Autodesk Inventor part; units mm, degrees
(part 10 of 11)
sketch "22" plane through (0, 0, 0) normal (0, 0, 1) x (1, 0, 0)
  line L0 (33.782, 19.812) -> (33.782, 30.7159)
  arc A0 (-2.032, 21.8669) -> (-2.032, 19.0271) centre (-2.032, 20.447) ccw
  arc A1 (-2.032, 19.0271) -> (-2.032, 21.8669) centre (-2.032, 20.447) ccw
  arc A2 (16.383, 40.2819) -> (16.383, 37.4421) centre (16.383, 38.862) ccw
  arc A3 (16.383, 37.4421) -> (16.383, 40.2819) centre (16.383, 38.862) ccw
  arc A4 (0.508, 19.8438) -> (0.508, 19.7803) centre (0.508, 19.812) ccw
  arc A5 (3.048, 19.7803) -> (3.048, 19.8438) centre (3.048, 19.812) ccw
  line L1 (0.508, 19.812) -> (3.048, 19.812)
  arc A6 (-0.7395, 21.1045) -> (-0.7845, 21.0595) centre (-0.762, 21.082) ccw
  arc A7 (0.4855, 19.7895) -> (0.5305, 19.8345) centre (0.508, 19.812) ccw
  line L2 (-0.762, 21.082) -> (0.508, 19.812)
  arc A8 (-2.0545, 19.8345) -> (-2.0095, 19.7895) centre (-2.032, 19.812) ccw
  arc A9 (-0.7395, 21.0595) -> (-0.7845, 21.1045) centre (-0.762, 21.082) ccw
  line L3 (-2.032, 19.812) -> (-0.762, 21.082)
  arc A10 (-0.7845, 18.5195) -> (-0.7395, 18.5645) centre (-0.762, 18.542) ccw
  arc A11 (-2.0095, 19.8345) -> (-2.0545, 19.7895) centre (-2.032, 19.812) ccw
  line L4 (-0.762, 18.542) -> (-2.032, 19.812)
  arc A12 (3.048, 18.5103) -> (3.048, 18.5738) centre (3.048, 18.542) ccw
  arc A13 (-0.762, 18.5738) -> (-0.762, 18.5102) centre (-0.762, 18.542) ccw
  line L5 (3.048, 18.542) -> (-0.762, 18.542)
  arc A14 (17.0498, 36.322) -> (16.9862, 36.322) centre (17.018, 36.322) ccw
  arc A15 (16.9862, 33.782) -> (17.0497, 33.782) centre (17.018, 33.782) ccw
  line L6 (17.018, 36.322) -> (17.018, 33.782)
  arc A16 (15.7705, 37.6145) -> (15.7255, 37.5695) centre (15.748, 37.592) ccw
  arc A17 (16.9955, 36.2995) -> (17.0405, 36.3445) centre (17.018, 36.322) ccw
  line L7 (15.748, 37.592) -> (17.018, 36.322)
  arc A18 (17.0405, 38.8395) -> (16.9955, 38.8845) centre (17.018, 38.862) ccw
  arc A19 (15.7255, 37.6145) -> (15.7705, 37.5695) centre (15.748, 37.592) ccw
  line L8 (17.018, 38.862) -> (15.748, 37.592)
  arc A20 (18.2655, 37.5695) -> (18.3105, 37.6145) centre (18.288, 37.592) ccw
  arc A21 (17.0405, 38.8845) -> (16.9955, 38.8395) centre (17.018, 38.862) ccw
  line L9 (18.288, 37.592) -> (17.018, 38.862)
  arc A22 (18.2563, 33.782) -> (18.3197, 33.782) centre (18.288, 33.782) ccw
  arc A23 (18.3198, 37.592) -> (18.2562, 37.592) centre (18.288, 37.592) ccw
  line L10 (18.288, 33.782) -> (18.288, 37.592)
  arc A24 (18.2563, 18.542) -> (18.3197, 18.542) centre (18.288, 18.542) ccw
  arc A25 (18.3197, 33.782) -> (18.2563, 33.782) centre (18.288, 33.782) ccw
  line L11 (18.288, 18.542) -> (18.288, 33.782)
  arc A26 (3.048, 18.5738) -> (3.048, 18.5103) centre (3.048, 18.542) ccw
  arc A27 (18.288, 18.5103) -> (18.288, 18.5738) centre (18.288, 18.542) ccw
  line L12 (3.048, 18.542) -> (18.288, 18.542)
  arc A28 (3.0162, 18.542) -> (3.0797, 18.542) centre (3.048, 18.542) ccw
  line L13 (3.048, 19.812) -> (3.048, 18.542)
  arc A29 (3.0797, 30.7159) -> (3.0162, 30.7159) centre (3.048, 30.7159) ccw
  arc A30 (3.0162, 19.812) -> (3.0797, 19.812) centre (3.048, 19.812) ccw
  line L14 (3.048, 30.7159) -> (3.048, 19.812)
  arc A31 (3.0162, 30.7159) -> (3.0797, 30.7159) centre (3.048, 30.7159) ccw
  line L15 (18.542, 3.048) -> (19.812, 3.048)
  arc A32 (19.812, 3.0162) -> (19.812, 3.0797) centre (19.812, 3.048) ccw
  arc A33 (18.542, 3.0797) -> (18.542, 3.0162) centre (18.542, 3.048) ccw
  line L16 (19.812, 3.048) -> (30.7159, 3.048)
  arc A34 (30.7159, 3.0162) -> (30.7159, 3.0797) centre (30.7159, 3.048) ccw
  arc A35 (19.812, 3.0797) -> (19.812, 3.0162) centre (19.812, 3.048) ccw
  arc A36 (6.1141, 33.7503) -> (6.1141, 33.8137) centre (6.1141, 33.782) ccw
  arc A37 (6.1141, 33.782) -> (3.048, 30.7159) centre (6.1141, 30.7159) ccw
  arc A38 (17.018, 33.7503) -> (17.018, 33.8137) centre (17.018, 33.782) ccw
  arc A39 (6.1141, 33.8137) -> (6.1141, 33.7503) centre (6.1141, 33.782) ccw
  line L17 (17.018, 33.782) -> (6.1141, 33.782)
  arc A40 (18.288, 33.7503) -> (18.288, 33.8137) centre (18.288, 33.782) ccw
  arc A41 (17.018, 33.8137) -> (17.018, 33.7503) centre (17.018, 33.782) ccw
  line L18 (18.288, 33.782) -> (17.018, 33.782)
  arc A42 (33.8137, 30.7159) -> (33.7503, 30.7159) centre (33.782, 30.7159) ccw
  arc A43 (20.447, 40.2819) -> (20.447, 37.4421) centre (20.447, 38.862) ccw
  arc A44 (20.447, 37.4421) -> (20.447, 40.2819) centre (20.447, 38.862) ccw
  arc A45 (38.862, 21.8669) -> (38.862, 19.0271) centre (38.862, 20.447) ccw
  arc A46 (38.862, 19.0271) -> (38.862, 21.8669) centre (38.862, 20.447) ccw
  arc A47 (19.8438, 36.322) -> (19.7803, 36.322) centre (19.812, 36.322) ccw
  arc A48 (19.7803, 33.782) -> (19.8438, 33.782) centre (19.812, 33.782) ccw
  line L19 (19.812, 36.322) -> (19.812, 33.782)
  arc A49 (21.1045, 37.5695) -> (21.0595, 37.6145) centre (21.082, 37.592) ccw
  arc A50 (19.7895, 36.3445) -> (19.8345, 36.2995) centre (19.812, 36.322) ccw
  line L20 (21.082, 37.592) -> (19.812, 36.322)
  arc A51 (19.8345, 38.8845) -> (19.7895, 38.8395) centre (19.812, 38.862) ccw
  arc A52 (21.0595, 37.5695) -> (21.1045, 37.6145) centre (21.082, 37.592) ccw
  line L21 (19.812, 38.862) -> (21.082, 37.592)
  arc A53 (18.5195, 37.6145) -> (18.5645, 37.5695) centre (18.542, 37.592) ccw
  arc A54 (19.8345, 38.8395) -> (19.7895, 38.8845) centre (19.812, 38.862) ccw
  line L22 (18.542, 37.592) -> (19.812, 38.862)
  arc A55 (18.5103, 33.782) -> (18.5738, 33.782) centre (18.542, 33.782) ccw
  arc A56 (18.5738, 37.592) -> (18.5102, 37.592) centre (18.542, 37.592) ccw
  line L23 (18.542, 33.782) -> (18.542, 37.592)
  arc A57 (36.322, 19.7803) -> (36.322, 19.8438) centre (36.322, 19.812) ccw
  arc A58 (33.782, 19.8438) -> (33.782, 19.7803) centre (33.782, 19.812) ccw
  line L24 (36.322, 19.812) -> (33.782, 19.812)
  arc A59 (37.6145, 21.0595) -> (37.5695, 21.1045) centre (37.592, 21.082) ccw
  arc A60 (36.2995, 19.8345) -> (36.3445, 19.7895) centre (36.322, 19.812) ccw
  line L25 (37.592, 21.082) -> (36.322, 19.812)
  arc A61 (38.8395, 19.7895) -> (38.8845, 19.8345) centre (38.862, 19.812) ccw
  arc A62 (37.6145, 21.1045) -> (37.5695, 21.0595) centre (37.592, 21.082) ccw
  line L26 (38.862, 19.812) -> (37.592, 21.082)
  arc A63 (37.5695, 18.5645) -> (37.6145, 18.5195) centre (37.592, 18.542) ccw
  arc A64 (33.7503, 19.812) -> (33.8137, 19.812) centre (33.782, 19.812) ccw
  arc A65 (38.8845, 19.7895) -> (38.8395, 19.8345) centre (38.862, 19.812) ccw
  line L27 (37.592, 18.542) -> (38.862, 19.812)
  arc A66 (33.782, 18.5738) -> (33.782, 18.5103) centre (33.782, 18.542) ccw
  arc A67 (37.592, 18.5102) -> (37.592, 18.5738) centre (37.592, 18.542) ccw
  line L28 (33.782, 18.542) -> (37.592, 18.542)
  arc A68 (18.542, 18.5738) -> (18.542, 18.5103) centre (18.542, 18.542) ccw
  arc A69 (33.782, 18.5103) -> (33.782, 18.5738) centre (33.782, 18.542) ccw
  line L29 (18.542, 18.542) -> (33.782, 18.542)
  arc A70 (18.5738, 33.782) -> (18.5103, 33.782) centre (18.542, 33.782) ccw
  arc A71 (18.5103, 18.542) -> (18.5738, 18.542) centre (18.542, 18.542) ccw
  line L30 (18.542, 33.782) -> (18.542, 18.542)
  arc A72 (19.812, 33.7503) -> (19.812, 33.8137) centre (19.812, 33.782) ccw
  arc A73 (18.542, 33.8137) -> (18.542, 33.7503) centre (18.542, 33.782) ccw
  line L31 (19.812, 33.782) -> (18.542, 33.782)
  arc A74 (30.7159, 33.7503) -> (30.7159, 33.8137) centre (30.7159, 33.782) ccw
  arc A75 (19.812, 33.8137) -> (19.812, 33.7503) centre (19.812, 33.782) ccw
  line L32 (30.7159, 33.782) -> (19.812, 33.782)
  arc A76 (30.7159, 33.8137) -> (30.7159, 33.7503) centre (30.7159, 33.782) ccw
  arc A77 (33.7503, 30.7159) -> (33.8137, 30.7159) centre (33.782, 30.7159) ccw
  arc A78 (33.782, 30.7159) -> (30.7159, 33.782) centre (30.7159, 30.7159) ccw
  arc A79 (3.0797, 19.812) -> (3.0162, 19.812) centre (3.048, 19.812) ccw
  arc A80 (33.7503, 18.542) -> (33.8137, 18.542) centre (33.782, 18.542) ccw
  arc A81 (33.8137, 19.812) -> (33.7503, 19.812) centre (33.782, 19.812) ccw
  line L33 (33.782, 18.542) -> (33.782, 19.812)
  arc A82 (38.862, 17.8029) -> (38.862, 14.9631) centre (38.862, 16.383) ccw
  line L34 (19.812, -2.032) -> (21.082, -0.762)
  arc A83 (21.1045, -0.7845) -> (21.0595, -0.7395) centre (21.082, -0.762) ccw
  arc A84 (19.7895, -2.0095) -> (19.8345, -2.0545) centre (19.812, -2.032) ccw
  line L35 (21.082, -0.762) -> (19.812, 0.508)
  arc A85 (3.0797, 18.288) -> (3.0162, 18.288) centre (3.048, 18.288) ccw
  arc A86 (19.8345, 0.5305) -> (19.7895, 0.4855) centre (19.812, 0.508) ccw
  arc A87 (21.0595, -0.7845) -> (21.1045, -0.7395) centre (21.082, -0.762) ccw
  line L36 (19.812, 0.508) -> (19.812, 3.048)
  arc A88 (19.8438, 3.048) -> (19.7803, 3.048) centre (19.812, 3.048) ccw
  arc A89 (19.7802, 0.508) -> (19.8438, 0.508) centre (19.812, 0.508) ccw
  line L37 (33.782, 18.288) -> (37.592, 18.288)
  arc A90 (37.592, 18.2563) -> (37.592, 18.3197) centre (37.592, 18.288) ccw
  arc A91 (33.782, 18.3197) -> (33.782, 18.2563) centre (33.782, 18.288) ccw
  line L38 (37.592, 18.288) -> (38.862, 17.018)
  arc A92 (38.8395, 16.9955) -> (38.8845, 17.0405) centre (38.862, 17.018) ccw
  arc A93 (37.6145, 18.3105) -> (37.5695, 18.2655) centre (37.592, 18.288) ccw
  line L39 (18.542, 18.288) -> (18.542, 3.048)
  arc A94 (18.5103, 3.048) -> (18.5738, 3.048) centre (18.542, 3.048) ccw
  arc A95 (18.5738, 18.288) -> (18.5103, 18.288) centre (18.542, 18.288) ccw
  line L40 (18.542, 3.048) -> (18.542, -0.762)
  arc A96 (18.5103, -0.762) -> (18.5738, -0.762) centre (18.542, -0.762) ccw
  arc A97 (18.5738, 3.048) -> (18.5103, 3.048) centre (18.542, 3.048) ccw
  line L41 (18.542, -0.762) -> (19.812, -2.032)
  arc A98 (19.7895, -2.0545) -> (19.8345, -2.0095) centre (19.812, -2.032) ccw
  arc A99 (18.5645, -0.7395) -> (18.5195, -0.7845) centre (18.542, -0.762) ccw
  line L42 (38.862, 17.018) -> (37.592, 15.748)
  arc A100 (37.5695, 15.7705) -> (37.6145, 15.7255) centre (37.592, 15.748) ccw
  line L43 (3.048, 18.288) -> (3.048, 17.018)
  arc A101 (3.0162, 17.018) -> (3.0797, 17.018) centre (3.048, 17.018) ccw
  arc A102 (30.7159, 3.048) -> (33.782, 6.1141) centre (30.7159, 6.1141) ccw
  arc A103 (30.7159, 3.0797) -> (30.7159, 3.0162) centre (30.7159, 3.048) ccw
  arc A104 (33.8137, 6.1141) -> (33.7503, 6.1141) centre (33.782, 6.1141) ccw
  line L44 (33.782, 6.1141) -> (33.782, 17.018)
  arc A105 (33.8137, 17.018) -> (33.7503, 17.018) centre (33.782, 17.018) ccw
  arc A106 (33.7503, 6.1141) -> (33.8137, 6.1141) centre (33.782, 6.1141) ccw
  line L45 (33.782, 17.018) -> (33.782, 18.288)
  arc A107 (33.8137, 18.288) -> (33.7503, 18.288) centre (33.782, 18.288) ccw
  arc A108 (33.7503, 17.018) -> (33.8137, 17.018) centre (33.782, 17.018) ccw
  line L46 (33.782, 18.288) -> (18.542, 18.288)
  arc A109 (18.542, 18.3197) -> (18.542, 18.2563) centre (18.542, 18.288) ccw
  arc A110 (33.782, 18.2563) -> (33.782, 18.3197) centre (33.782, 18.288) ccw
  arc A111 (38.862, 14.9631) -> (38.862, 17.8029) centre (38.862, 16.383) ccw
  line L47 (3.048, 17.018) -> (3.048, 6.1141)
  arc A112 (3.0162, 6.1141) -> (3.0797, 6.1141) centre (3.048, 6.1141) ccw
  arc A113 (3.0797, 17.018) -> (3.0162, 17.018) centre (3.048, 17.018) ccw
  arc A114 (3.048, 6.1141) -> (6.1141, 3.048) centre (6.1141, 6.1141) ccw
  arc A115 (3.0797, 6.1141) -> (3.0162, 6.1141) centre (3.048, 6.1141) ccw
  arc A116 (6.1141, 3.0162) -> (6.1141, 3.0797) centre (6.1141, 3.048) ccw
  line L48 (6.1141, 3.048) -> (17.018, 3.048)
  arc A117 (17.018, 3.0162) -> (17.018, 3.0797) centre (17.018, 3.048) ccw
  arc A118 (6.1141, 3.0797) -> (6.1141, 3.0162) centre (6.1141, 3.048) ccw
  line L49 (17.018, 3.048) -> (18.288, 3.048)
  arc A119 (18.288, 3.0162) -> (18.288, 3.0797) centre (18.288, 3.048) ccw
  arc A120 (17.018, 3.0797) -> (17.018, 3.0162) centre (17.018, 3.048) ccw
  line L50 (18.288, 3.048) -> (18.288, 18.288)
  arc A121 (18.3197, 18.288) -> (18.2563, 18.288) centre (18.288, 18.288) ccw
  arc A122 (18.2563, 3.048) -> (18.3197, 3.048) centre (18.288, 3.048) ccw
  line L51 (18.288, 18.288) -> (3.048, 18.288)
  arc A123 (3.048, 18.3197) -> (3.048, 18.2563) centre (3.048, 18.288) ccw
  arc A124 (18.288, 18.2563) -> (18.288, 18.3197) centre (18.288, 18.288) ccw
  line L52 (3.048, 18.288) -> (-0.762, 18.288)
  arc A125 (-0.762, 18.3197) -> (-0.762, 18.2563) centre (-0.762, 18.288) ccw
  arc A126 (3.048, 18.2563) -> (3.048, 18.3197) centre (3.048, 18.288) ccw
  line L53 (-0.762, 18.288) -> (-2.032, 17.018)
  arc A127 (-2.0545, 17.0405) -> (-2.0095, 16.9955) centre (-2.032, 17.018) ccw
  arc A128 (-0.7395, 18.2655) -> (-0.7845, 18.3105) centre (-0.762, 18.288) ccw
  line L54 (-2.032, 17.018) -> (-0.762, 15.748)
  arc A129 (-0.7845, 15.7255) -> (-0.7395, 15.7705) centre (-0.762, 15.748) ccw
  arc A130 (-2.0095, 17.0405) -> (-2.0545, 16.9955) centre (-2.032, 17.018) ccw
  line L55 (-0.762, 15.748) -> (0.508, 17.018)
  arc A131 (0.5305, 16.9955) -> (0.4855, 17.0405) centre (0.508, 17.018) ccw
  arc A132 (-0.7845, 15.7705) -> (-0.7395, 15.7255) centre (-0.762, 15.748) ccw
  line L56 (0.508, 17.018) -> (3.048, 17.018)
  arc A133 (3.048, 16.9862) -> (3.048, 17.0497) centre (3.048, 17.018) ccw
  arc A134 (0.508, 17.0498) -> (0.508, 16.9862) centre (0.508, 17.018) ccw
  line L57 (18.288, 3.048) -> (18.288, -0.762)
  arc A135 (18.2563, -0.762) -> (18.3197, -0.762) centre (18.288, -0.762) ccw
  arc A136 (18.3197, 3.048) -> (18.2563, 3.048) centre (18.288, 3.048) ccw
  line L58 (18.288, -0.762) -> (17.018, -2.032)
  arc A137 (38.8845, 16.9955) -> (38.8395, 17.0405) centre (38.862, 17.018) ccw
  arc A138 (16.9955, -2.0095) -> (17.0405, -2.0545) centre (17.018, -2.032) ccw
  arc A139 (18.3105, -0.7845) -> (18.2655, -0.7395) centre (18.288, -0.762) ccw
  line L59 (17.018, -2.032) -> (15.748, -0.762)
  arc A140 (15.7705, -0.7395) -> (15.7255, -0.7845) centre (15.748, -0.762) ccw
  arc A141 (16.9955, -2.0545) -> (17.0405, -2.0095) centre (17.018, -2.032) ccw
  line L60 (15.748, -0.762) -> (17.018, 0.508)
  arc A142 (17.0405, 0.4855) -> (16.9955, 0.5305) centre (17.018, 0.508) ccw
  arc A143 (15.7255, -0.7395) -> (15.7705, -0.7845) centre (15.748, -0.762) ccw
  line L61 (17.018, 0.508) -> (17.018, 3.048)
  arc A144 (17.0498, 3.048) -> (16.9862, 3.048) centre (17.018, 3.048) ccw
  arc A145 (16.9862, 0.508) -> (17.0498, 0.508) centre (17.018, 0.508) ccw
  arc A146 (-2.032, 14.9631) -> (-2.032, 17.8029) centre (-2.032, 16.383) ccw
  arc A147 (-2.032, 17.8029) -> (-2.032, 14.9631) centre (-2.032, 16.383) ccw
  arc A148 (16.383, -3.4519) -> (16.383, -0.6121) centre (16.383, -2.032) ccw
  arc A149 (16.383, -0.6121) -> (16.383, -3.4519) centre (16.383, -2.032) ccw
  line L62 (37.592, 15.748) -> (36.322, 17.018)
  arc A150 (36.3445, 17.0405) -> (36.2995, 16.9955) centre (36.322, 17.018) ccw
  arc A151 (37.5695, 15.7255) -> (37.6145, 15.7705) centre (37.592, 15.748) ccw
  line L63 (36.322, 17.018) -> (33.782, 17.018)
  arc A152 (33.782, 17.0498) -> (33.782, 16.9862) centre (33.782, 17.018) ccw
  arc A153 (36.322, 16.9862) -> (36.322, 17.0498) centre (36.322, 17.018) ccw
  arc A154 (20.447, -3.4519) -> (20.447, -0.6121) centre (20.447, -2.032) ccw
  arc A155 (20.447, -0.6121) -> (20.447, -3.4519) centre (20.447, -2.032) ccw
  constraints: 440 point on circle, 156 centre point, 128 end point, 88 point on line
sketch "25" plane through (0, 0, 0) normal (0, 0, 1) x (1, 0, 0)
  arc A0 (12.1564, 34.6207) -> (12.131, 34.6207) centre (12.1437, 34.6207) ccw
  line L0 (12.1437, 34.0614) -> (12.1437, 34.6207)
  arc A1 (11.862, 34.2351) -> (11.862, 34.2605) centre (11.862, 34.2478) ccw
  arc A2 (11.5824, 34.2605) -> (11.5824, 34.2351) centre (11.5824, 34.2478) ccw
  line L1 (11.862, 34.2478) -> (11.5824, 34.2478)
  arc A3 (11.9642, 34.3321) -> (11.9463, 34.35) centre (11.9553, 34.341) ccw
  arc A4 (13.4527, 34.3537) -> (13.4527, 34.3283) centre (13.4527, 34.341) ccw
  line L2 (13.6392, 34.341) -> (13.4527, 34.341)
  arc A5 (13.6265, 34.1546) -> (13.6519, 34.1546) centre (13.6392, 34.1546) ccw
  arc A6 (33.6734, 12.9789) -> (33.6464, 13.0059) centre (33.6599, 12.9924) ccw
  line L3 (33.5031, 12.8356) -> (33.6599, 12.9924)
  arc A7 (33.1896, 12.8547) -> (33.1896, 12.8166) centre (33.1896, 12.8356) ccw
  arc A8 (33.5031, 12.8166) -> (33.5031, 12.8547) centre (33.5031, 12.8356) ccw
  line L4 (33.1896, 12.8356) -> (33.5031, 12.8356)
  arc A9 (32.8895, 13.1626) -> (32.8626, 13.1357) centre (32.8761, 13.1492) ccw
  arc A10 (33.1761, 12.8221) -> (33.2031, 12.8491) centre (33.1896, 12.8356) ccw
  line L5 (32.8761, 13.1491) -> (33.1896, 12.8356)
  arc A11 (32.7363, 13.4712) -> (32.7022, 13.4542) centre (32.7193, 13.4627) ccw
  arc A12 (13.6519, 34.341) -> (13.6265, 34.341) centre (13.6392, 34.341) ccw
  line L6 (13.6392, 34.1546) -> (13.6392, 34.341)
  arc A13 (13.537, 34.0704) -> (13.5549, 34.0524) centre (13.546, 34.0614) ccw
  arc A14 (13.6481, 34.1456) -> (13.6302, 34.1636) centre (13.6392, 34.1546) ccw
  line L7 (13.546, 34.0614) -> (13.6392, 34.1546)
  arc A15 (13.3595, 34.0741) -> (13.3595, 34.0487) centre (13.3595, 34.0614) ccw
  arc A16 (13.546, 34.0487) -> (13.546, 34.0741) centre (13.546, 34.0614) ccw
  line L8 (13.3595, 34.0614) -> (13.546, 34.0614)
  arc A17 (13.3506, 34.0524) -> (13.3685, 34.0704) centre (13.3595, 34.0614) ccw
  line L9 (13.2663, 34.1546) -> (13.3595, 34.0614)
  arc A18 (13.279, 34.5275) -> (13.2536, 34.5275) centre (13.2663, 34.5275) ccw
  arc A19 (13.2536, 34.1546) -> (13.279, 34.1546) centre (13.2663, 34.1546) ccw
  line L10 (13.2663, 34.5275) -> (13.2663, 34.1546)
  arc A20 (13.3685, 34.6117) -> (13.3506, 34.6296) centre (13.3595, 34.6207) ccw
  arc A21 (13.2574, 34.5364) -> (13.2753, 34.5185) centre (13.2663, 34.5275) ccw
  line L11 (13.3595, 34.6207) -> (13.2663, 34.5275)
  arc A22 (13.546, 34.608) -> (13.546, 34.6334) centre (13.546, 34.6207) ccw
  arc A23 (13.3595, 34.6334) -> (13.3595, 34.608) centre (13.3595, 34.6207) ccw
  line L12 (13.546, 34.6207) -> (13.3595, 34.6207)
  arc A24 (13.6302, 34.5185) -> (13.6482, 34.5364) centre (13.6392, 34.5275) ccw
  arc A25 (13.5549, 34.6296) -> (13.537, 34.6117) centre (13.546, 34.6207) ccw
  line L13 (13.6392, 34.5275) -> (13.546, 34.6207)
  arc A26 (13.0689, 34.5185) -> (13.0868, 34.5364) centre (13.0779, 34.5275) ccw
  arc A27 (12.9936, 34.6296) -> (12.9757, 34.6117) centre (12.9846, 34.6207) ccw
  line L14 (13.0779, 34.5275) -> (12.9847, 34.6207)
  arc A28 (13.0652, 34.1546) -> (13.0906, 34.1546) centre (13.0779, 34.1546) ccw
  arc A29 (13.0906, 34.5275) -> (13.0652, 34.5275) centre (13.0779, 34.5275) ccw
  line L15 (13.0779, 34.1546) -> (13.0779, 34.5275)
  arc A30 (12.9757, 34.0704) -> (12.9936, 34.0524) centre (12.9846, 34.0614) ccw
  arc A31 (13.0868, 34.1456) -> (13.0689, 34.1636) centre (13.0779, 34.1546) ccw
  line L16 (12.9846, 34.0614) -> (13.0779, 34.1546)
  arc A32 (12.7982, 34.0741) -> (12.7982, 34.0487) centre (12.7982, 34.0614) ccw
  line L17 (12.7982, 34.0614) -> (12.9846, 34.0614)
  arc A33 (11.8531, 34.2568) -> (11.871, 34.2388) centre (11.862, 34.2478) ccw
  line L18 (11.9552, 34.341) -> (11.862, 34.2478)
  arc A34 (11.9679, 34.5275) -> (11.9425, 34.5275) centre (11.9552, 34.5275) ccw
  arc A35 (32.859, 13.1406) -> (32.8931, 13.1577) centre (32.8761, 13.1492) ccw
  line L19 (32.7193, 13.4627) -> (32.8761, 13.1491)
  arc A36 (33.6464, 12.3569) -> (33.6734, 12.3839) centre (33.6599, 12.3704) ccw
  arc A37 (33.5166, 12.5406) -> (33.4897, 12.5137) centre (33.5031, 12.5272) ccw
  line L20 (33.6599, 12.3704) -> (33.5031, 12.5272)
  arc A38 (33.6408, 12.0569) -> (33.6789, 12.0569) centre (33.6599, 12.0569) ccw
  arc A39 (33.6789, 12.3704) -> (33.6409, 12.3704) centre (33.6599, 12.3704) ccw
  line L21 (33.6599, 12.0569) -> (33.6599, 12.3704)
  arc A40 (33.4897, 11.9136) -> (33.5166, 11.8866) centre (33.5031, 11.9001) ccw
  arc A41 (33.6734, 12.0434) -> (33.6464, 12.0703) centre (33.6599, 12.0569) ccw
  line L22 (33.5031, 11.9001) -> (33.6599, 12.0569)
  arc A42 (32.8761, 11.9192) -> (32.8761, 11.8811) centre (32.8761, 11.9001) ccw
  arc A43 (33.5031, 11.881) -> (33.5031, 11.9191) centre (33.5031, 11.9001) ccw
  line L23 (32.8761, 11.9001) -> (33.5031, 11.9001)
  arc A44 (32.7328, 12.0703) -> (32.7058, 12.0434) centre (32.7193, 12.0569) ccw
  arc A45 (32.8626, 11.8867) -> (32.8895, 11.9136) centre (32.8761, 11.9001) ccw
  line L24 (32.7193, 12.0569) -> (32.8761, 11.9001)
  arc A46 (32.7383, 12.3704) -> (32.7002, 12.3704) centre (32.7193, 12.3704) ccw
  arc A47 (32.7002, 12.0569) -> (32.7384, 12.0569) centre (32.7193, 12.0569) ccw
  line L25 (32.7193, 12.3704) -> (32.7193, 12.0569)
  arc A48 (32.8895, 12.5137) -> (32.8626, 12.5406) centre (32.8761, 12.5272) ccw
  arc A49 (32.7058, 12.3839) -> (32.7328, 12.3569) centre (32.7193, 12.3704) ccw
  line L26 (32.8761, 12.5272) -> (32.7193, 12.3704)
  arc A50 (17.6429, 33.1576) -> (17.6699, 33.1846) centre (17.6564, 33.1711) ccw
  arc A51 (17.5131, 33.3413) -> (17.4861, 33.3144) centre (17.4996, 33.3278) ccw
  line L27 (17.6564, 33.1711) -> (17.4996, 33.3279)
  arc A52 (17.9699, 33.152) -> (17.9699, 33.1901) centre (17.9699, 33.1711) ccw
  arc A53 (17.6564, 33.1901) -> (17.6564, 33.152) centre (17.6564, 33.1711) ccw
  line L28 (17.9699, 33.1711) -> (17.6564, 33.1711)
  arc A54 (18.1401, 33.3144) -> (18.1132, 33.3413) centre (18.1267, 33.3279) ccw
  arc A55 (17.9565, 33.1846) -> (17.9834, 33.1576) centre (17.9699, 33.1711) ccw
  line L29 (18.1267, 33.3279) -> (17.9699, 33.1711)
  arc A56 (18.1457, 33.6414) -> (18.1076, 33.6414) centre (18.1267, 33.6414) ccw
  arc A57 (18.1076, 33.3279) -> (18.1457, 33.3279) centre (18.1267, 33.3279) ccw
  line L30 (18.1267, 33.6414) -> (18.1267, 33.3279)
  arc A58 (17.9834, 33.8116) -> (17.9565, 33.7847) centre (17.9699, 33.7982) ccw
  arc A59 (18.1132, 33.6279) -> (18.1401, 33.6549) centre (18.1267, 33.6414) ccw
  line L31 (17.9699, 33.7982) -> (18.1267, 33.6414)
  arc A60 (17.8131, 33.8172) -> (17.8131, 33.7791) centre (17.8131, 33.7982) ccw
  arc A61 (17.9699, 33.7791) -> (17.9699, 33.8172) centre (17.9699, 33.7982) ccw
  line L32 (17.8131, 33.7982) -> (17.9699, 33.7982)
  arc A62 (17.4911, 33.6584) -> (17.5081, 33.6244) centre (17.4996, 33.6414) ccw
  arc A63 (17.8217, 33.7811) -> (17.8046, 33.8152) centre (17.8132, 33.7982) ccw
  line L33 (17.4996, 33.6414) -> (17.8131, 33.7982)
  arc A64 (17.5187, 34.1117) -> (17.4806, 34.1117) centre (17.4996, 34.1117) ccw
  arc A65 (17.4806, 33.6414) -> (17.5187, 33.6414) centre (17.4996, 33.6414) ccw
  line L34 (17.4996, 34.1117) -> (17.4996, 33.6414)
  arc A66 (18.1267, 34.0926) -> (18.1267, 34.1307) centre (18.1267, 34.1117) ccw
  arc A67 (17.4996, 34.1307) -> (17.4996, 34.0926) centre (17.4996, 34.1117) ccw
  line L35 (18.1267, 34.1117) -> (17.4996, 34.1117)
  arc A68 (17.0209, 33.1846) -> (17.0479, 33.1576) centre (17.0344, 33.1711) ccw
  arc A69 (17.2046, 33.3144) -> (17.1777, 33.3413) centre (17.1912, 33.3278) ccw
  line L36 (17.0344, 33.1711) -> (17.1912, 33.3279)
  arc A70 (16.7209, 33.1901) -> (16.7209, 33.152) centre (16.7209, 33.1711) ccw
  arc A71 (17.0344, 33.152) -> (17.0344, 33.1901) centre (17.0344, 33.1711) ccw
  line L37 (16.7209, 33.1711) -> (17.0344, 33.1711)
  arc A72 (16.5776, 33.3413) -> (16.5506, 33.3144) centre (16.5641, 33.3279) ccw
  arc A73 (16.7074, 33.1576) -> (16.7343, 33.1846) centre (16.7209, 33.1711) ccw
  line L38 (16.5641, 33.3279) -> (16.7209, 33.1711)
  arc A74 (16.5832, 33.9549) -> (16.5451, 33.9549) centre (16.5641, 33.9549) ccw
  arc A75 (16.5451, 33.3279) -> (16.5832, 33.3279) centre (16.5641, 33.3279) ccw
  line L39 (16.5641, 33.9549) -> (16.5641, 33.3279)
  arc A76 (16.7343, 34.0982) -> (16.7074, 34.1252) centre (16.7209, 34.1117) ccw
  arc A77 (16.5506, 33.9684) -> (16.5776, 33.9414) centre (16.5641, 33.9549) ccw
  line L40 (16.7209, 34.1117) -> (16.5641, 33.9549)
  arc A78 (17.0344, 34.0926) -> (17.0344, 34.1307) centre (17.0344, 34.1117) ccw
  arc A79 (16.7209, 34.1307) -> (16.7209, 34.0926) centre (16.7209, 34.1117) ccw
  line L41 (17.0344, 34.1117) -> (16.7209, 34.1117)
  arc A80 (17.1777, 33.9415) -> (17.2046, 33.9684) centre (17.1912, 33.9549) ccw
  arc A81 (17.0479, 34.1252) -> (17.0209, 34.0982) centre (17.0344, 34.1117) ccw
  line L42 (17.1912, 33.9549) -> (17.0344, 34.1117)
  arc A82 (8.6096, 27.3105) -> (8.6096, 27.2724) centre (8.6096, 27.2914) ccw
  arc A83 (9.2367, 27.2724) -> (9.2367, 27.3105) centre (9.2367, 27.2914) ccw
  arc A84 (13.2753, 34.1636) -> (13.2574, 34.1456) centre (13.2663, 34.1546) ccw
  arc A85 (9.0934, 27.7482) -> (9.0665, 27.7752) centre (9.0799, 27.7617) ccw
  arc A86 (8.5961, 27.3049) -> (8.6231, 27.2779) centre (8.6096, 27.2914) ccw
  line L43 (9.0799, 27.7617) -> (8.6096, 27.2914)
  arc A87 (9.0609, 26.8211) -> (9.099, 26.8211) centre (9.0799, 26.8211) ccw
  arc A88 (9.099, 27.7617) -> (9.0609, 27.7617) centre (9.0799, 27.7617) ccw
  line L44 (9.0799, 26.8211) -> (9.0799, 27.7617)
  arc A89 (8.1309, 26.8346) -> (8.1579, 26.8076) centre (8.1444, 26.8211) ccw
  arc A90 (8.3146, 26.9644) -> (8.2877, 26.9913) centre (8.3012, 26.9778) ccw
  line L45 (8.1444, 26.8211) -> (8.3012, 26.9779)
  arc A91 (7.8309, 26.8401) -> (7.8309, 26.802) centre (7.8309, 26.8211) ccw
  arc A92 (8.1444, 26.802) -> (8.1444, 26.8401) centre (8.1444, 26.8211) ccw
  line L46 (7.8309, 26.8211) -> (8.1444, 26.8211)
  arc A93 (7.6876, 26.9913) -> (7.6606, 26.9644) centre (7.6741, 26.9779) ccw
  arc A94 (7.8174, 26.8076) -> (7.8443, 26.8346) centre (7.8309, 26.8211) ccw
  line L47 (7.6741, 26.9779) -> (7.8309, 26.8211)
  arc A95 (7.6932, 27.6049) -> (7.6551, 27.6049) centre (7.6741, 27.6049) ccw
  arc A96 (7.6551, 26.9779) -> (7.6932, 26.9779) centre (7.6741, 26.9779) ccw
  line L48 (7.6741, 27.6049) -> (7.6741, 26.9779)
  arc A97 (7.8443, 27.7482) -> (7.8174, 27.7752) centre (7.8309, 27.7617) ccw
  arc A98 (7.6606, 27.6184) -> (7.6876, 27.5914) centre (7.6741, 27.6049) ccw
  line L49 (7.8309, 27.7617) -> (7.6741, 27.6049)
  arc A99 (8.1444, 27.7426) -> (8.1444, 27.7807) centre (8.1444, 27.7617) ccw
  arc A100 (7.8309, 27.7807) -> (7.8309, 27.7426) centre (7.8309, 27.7617) ccw
  line L50 (8.1444, 27.7617) -> (7.8309, 27.7617)
  arc A101 (8.2877, 27.5915) -> (8.3146, 27.6184) centre (8.3012, 27.6049) ccw
  arc A102 (8.1579, 27.7752) -> (8.1309, 27.7482) centre (8.1444, 27.7617) ccw
  line L51 (8.3012, 27.6049) -> (8.1444, 27.7617)
  arc A103 (12.5255, 34.3321) -> (12.5076, 34.35) centre (12.5165, 34.341) ccw
  line L52 (12.4233, 34.2478) -> (12.1437, 34.2478)
  arc A104 (12.1437, 34.2605) -> (12.1437, 34.2351) centre (12.1437, 34.2478) ccw
  arc A105 (12.714, 34.1636) -> (12.696, 34.1456) centre (12.705, 34.1546) ccw
  arc A106 (11.9425, 34.341) -> (11.9679, 34.341) centre (11.9552, 34.341) ccw
  line L53 (11.9552, 34.5275) -> (11.9552, 34.341)
  arc A107 (11.871, 34.6297) -> (11.8531, 34.6117) centre (11.862, 34.6207) ccw
  arc A108 (11.9463, 34.5185) -> (11.9642, 34.5364) centre (11.9553, 34.5275) ccw
  line L54 (11.862, 34.6207) -> (11.9552, 34.5275)
  arc A109 (11.5824, 34.6334) -> (11.5824, 34.608) centre (11.5824, 34.6207) ccw
  arc A110 (11.862, 34.608) -> (11.862, 34.6334) centre (11.862, 34.6207) ccw
  line L55 (11.5824, 34.6207) -> (11.862, 34.6207)
  arc A111 (11.5697, 34.0614) -> (11.5951, 34.0614) centre (11.5824, 34.0614) ccw
  arc A112 (12.7893, 34.0524) -> (12.8072, 34.0704) centre (12.7982, 34.0614) ccw
  line L56 (12.705, 34.1546) -> (12.7982, 34.0614)
  arc A113 (12.7177, 34.5275) -> (12.6923, 34.5275) centre (12.705, 34.5275) ccw
  arc A114 (12.6923, 34.1546) -> (12.7177, 34.1546) centre (12.705, 34.1546) ccw
  line L57 (12.705, 34.5275) -> (12.705, 34.1546)
  arc A115 (12.8072, 34.6117) -> (12.7893, 34.6296) centre (12.7982, 34.6207) ccw
  arc A116 (11.5951, 34.6207) -> (11.5697, 34.6207) centre (11.5824, 34.6207) ccw
  line L58 (11.5824, 34.0614) -> (11.5824, 34.6207)
  arc A117 (12.5293, 34.5275) -> (12.5039, 34.5275) centre (12.5166, 34.5275) ccw
  line L59 (12.5166, 34.341) -> (12.4233, 34.2478)
  arc A118 (12.4144, 34.2568) -> (12.4323, 34.2388) centre (12.4234, 34.2478) ccw
  arc A119 (12.5039, 34.341) -> (12.5293, 34.341) centre (12.5166, 34.341) ccw
  line L60 (12.5166, 34.5275) -> (12.5166, 34.341)
  arc A120 (12.4323, 34.6297) -> (12.4144, 34.6117) centre (12.4234, 34.6207) ccw
  arc A121 (33.2086, 13.3059) -> (33.1705, 13.3059) centre (33.1896, 13.3059) ccw
  arc A122 (33.1705, 12.8356) -> (33.2086, 12.8356) centre (33.1896, 12.8356) ccw
  line L61 (33.1896, 13.3059) -> (33.1896, 12.8356)
  arc A123 (33.3598, 13.4492) -> (33.3329, 13.4761) centre (33.3464, 13.4627) ccw
  arc A124 (12.696, 34.5364) -> (12.714, 34.5185) centre (12.705, 34.5275) ccw
  line L62 (12.7982, 34.6207) -> (12.705, 34.5275)
  arc A125 (12.9847, 34.608) -> (12.9847, 34.6334) centre (12.9847, 34.6207) ccw
  arc A126 (12.7982, 34.6334) -> (12.7982, 34.608) centre (12.7982, 34.6207) ccw
  line L63 (12.9847, 34.6207) -> (12.7982, 34.6207)
  arc A127 (12.3391, 34.2568) -> (12.3212, 34.2388) centre (12.3301, 34.2478) ccw
  arc A128 (12.5076, 34.0524) -> (12.5255, 34.0704) centre (12.5166, 34.0614) ccw
  line L64 (12.3301, 34.2478) -> (12.5166, 34.0614)
  arc A129 (12.4233, 34.2351) -> (12.4233, 34.2605) centre (12.4233, 34.2478) ccw
  arc A130 (12.5076, 34.5185) -> (12.5255, 34.5364) centre (12.5165, 34.5275) ccw
  line L65 (12.4233, 34.6207) -> (12.5166, 34.5275)
  arc A131 (12.1437, 34.6334) -> (12.1437, 34.608) centre (12.1437, 34.6207) ccw
  arc A132 (12.4233, 34.608) -> (12.4233, 34.6334) centre (12.4233, 34.6207) ccw
  line L66 (12.1437, 34.6207) -> (12.4233, 34.6207)
  arc A133 (12.131, 34.0614) -> (12.1564, 34.0614) centre (12.1437, 34.0614) ccw
  arc A134 (33.5166, 13.4761) -> (33.4897, 13.4492) centre (33.5031, 13.4627) ccw
  line L67 (33.6599, 13.3059) -> (33.5031, 13.4627)
  arc A135 (33.6409, 12.9924) -> (33.679, 12.9924) centre (33.6599, 12.9924) ccw
  arc A136 (33.679, 13.3059) -> (33.6409, 13.3059) centre (33.6599, 13.3059) ccw
  line L68 (33.6599, 12.9924) -> (33.6599, 13.3059)
  arc A137 (33.4897, 12.8491) -> (33.5166, 12.8221) centre (33.5031, 12.8356) ccw
  arc A138 (12.9846, 34.0487) -> (12.9846, 34.0741) centre (12.9846, 34.0614) ccw
  arc A139 (13.6392, 34.3283) -> (13.6392, 34.3537) centre (13.6392, 34.341) ccw
  arc A140 (33.1761, 13.3194) -> (33.2031, 13.2925) centre (33.1896, 13.3059) ccw
  line L69 (33.3464, 13.4627) -> (33.1896, 13.3059)
  arc A141 (33.5031, 13.4436) -> (33.5031, 13.4817) centre (33.5031, 13.4627) ccw
  arc A142 (33.3464, 13.4817) -> (33.3464, 13.4436) centre (33.3464, 13.4627) ccw
  line L70 (33.5031, 13.4627) -> (33.3464, 13.4627)
  arc A143 (33.6464, 13.2925) -> (33.6734, 13.3194) centre (33.6599, 13.3059) ccw
  line L71 (8.6096, 27.2914) -> (9.2367, 27.2914)
  constraints: 344 point on circle, 144 centre point, 144 end point, 51 point on line
sketch "26" plane through (0, 0, 0) normal (0, 0, 1) x (1, 0, 0)
  line L0 (23.3846, 33.9861) -> (22.8683, 33.9861)
  arc A0 (22.8683, 34.0051) -> (22.8683, 33.967) centre (22.8683, 33.9861) ccw
  arc A1 (23.3846, 33.967) -> (23.3846, 34.0051) centre (23.3846, 33.9861) ccw
  line L1 (22.0856, 34.7606) -> (22.6019, 34.7606)
  arc A2 (22.6019, 34.7415) -> (22.6019, 34.7796) centre (22.6019, 34.7606) ccw
  arc A3 (22.0856, 34.7796) -> (22.0856, 34.7415) centre (22.0856, 34.7606) ccw
  line L2 (22.6019, 34.7606) -> (22.6019, 34.3733)
  arc A4 (22.5828, 34.3733) -> (22.6209, 34.3733) centre (22.6019, 34.3733) ccw
  arc A5 (22.6209, 34.7606) -> (22.5828, 34.7606) centre (22.6019, 34.7606) ccw
  line L3 (22.6019, 34.3733) -> (22.3437, 34.5024)
  arc A6 (22.3523, 34.5194) -> (22.3352, 34.4854) centre (22.3437, 34.5024) ccw
  arc A7 (22.5934, 34.3563) -> (22.6104, 34.3904) centre (22.6019, 34.3733) ccw
  line L4 (22.3437, 34.5024) -> (22.2147, 34.5024)
  arc A8 (22.2147, 34.5214) -> (22.2147, 34.4833) centre (22.2147, 34.5024) ccw
  arc A9 (22.3437, 34.4833) -> (22.3437, 34.5214) centre (22.3437, 34.5024) ccw
  line L5 (22.2147, 34.5024) -> (22.0856, 34.3733)
  arc A10 (22.0721, 34.3868) -> (22.0991, 34.3599) centre (22.0856, 34.3733) ccw
  arc A11 (22.2281, 34.4889) -> (22.2012, 34.5159) centre (22.2147, 34.5024) ccw
  line L6 (22.0856, 34.3733) -> (22.0856, 34.1152)
  arc A12 (22.0665, 34.1152) -> (22.1046, 34.1152) centre (22.0856, 34.1152) ccw
  arc A13 (22.1046, 34.3733) -> (22.0665, 34.3733) centre (22.0856, 34.3733) ccw
  line L7 (22.0856, 34.1152) -> (22.2147, 33.9861)
  arc A14 (22.2012, 33.9726) -> (22.2281, 33.9996) centre (22.2147, 33.9861) ccw
  arc A15 (22.0991, 34.1286) -> (22.0721, 34.1017) centre (22.0856, 34.1152) ccw
  line L8 (22.2147, 33.9861) -> (22.4728, 33.9861)
  arc A16 (22.4728, 33.967) -> (22.4728, 34.0051) centre (22.4728, 33.9861) ccw
  arc A17 (22.2147, 34.0051) -> (22.2147, 33.967) centre (22.2147, 33.9861) ccw
  line L9 (22.4728, 33.9861) -> (22.6019, 34.1152)
  arc A18 (22.6154, 34.1017) -> (22.5884, 34.1286) centre (22.6019, 34.1152) ccw
  arc A19 (22.4593, 33.9996) -> (22.4863, 33.9726) centre (22.4728, 33.9861) ccw
  line L10 (28.6676, 32.7111) -> (28.6676, 33.4856)
  arc A20 (28.6866, 33.4856) -> (28.6485, 33.4856) centre (28.6676, 33.4856) ccw
  arc A21 (28.6485, 32.7111) -> (28.6866, 32.7111) centre (28.6676, 32.7111) ccw
  line L11 (28.6676, 33.4856) -> (28.2803, 33.4856)
  arc A22 (28.2803, 33.5046) -> (28.2803, 33.4665) centre (28.2803, 33.4856) ccw
  arc A23 (28.6676, 33.4665) -> (28.6676, 33.5046) centre (28.6676, 33.4856) ccw
  line L12 (28.2803, 33.4856) -> (28.1513, 33.3565)
  arc A24 (28.1378, 33.37) -> (28.1647, 33.343) centre (28.1513, 33.3565) ccw
  arc A25 (28.2938, 33.4721) -> (28.2669, 33.499) centre (28.2803, 33.4856) ccw
  line L13 (28.1513, 33.3565) -> (28.1513, 33.0983)
  arc A26 (28.1322, 33.0983) -> (28.1703, 33.0983) centre (28.1513, 33.0983) ccw
  arc A27 (28.1703, 33.3565) -> (28.1322, 33.3565) centre (28.1513, 33.3565) ccw
  line L14 (28.1513, 33.0983) -> (28.2803, 32.9693)
  arc A28 (28.2669, 32.9558) -> (28.2938, 32.9827) centre (28.2803, 32.9693) ccw
  arc A29 (28.1647, 33.1118) -> (28.1378, 33.0848) centre (28.1513, 33.0983) ccw
  line L15 (28.2803, 32.9693) -> (28.6676, 32.9693)
  arc A30 (28.6676, 32.9502) -> (28.6676, 32.9883) centre (28.6676, 32.9693) ccw
  arc A31 (28.2803, 32.9883) -> (28.2803, 32.9502) centre (28.2803, 32.9693) ccw
  line L16 (28.4094, 32.9693) -> (28.1513, 32.7111)
  arc A32 (28.1378, 32.7246) -> (28.1647, 32.6976) centre (28.1513, 32.7111) ccw
  arc A33 (28.4229, 32.9558) -> (28.396, 32.9827) centre (28.4094, 32.9693) ccw
  line L17 (27.4977, 32.7111) -> (27.7558, 32.7111)
  arc A34 (27.7558, 32.6921) -> (27.7558, 32.7302) centre (27.7558, 32.7111) ccw
  arc A35 (27.4977, 32.7302) -> (27.4977, 32.6921) centre (27.4977, 32.7111) ccw
  line L18 (27.7558, 32.7111) -> (27.8849, 32.8402)
  arc A36 (27.8983, 32.8267) -> (27.8714, 32.8537) centre (27.8849, 32.8402) ccw
  arc A37 (27.7424, 32.7246) -> (27.7693, 32.6976) centre (27.7558, 32.7111) ccw
  line L19 (27.8849, 32.8402) -> (27.8849, 33.0983)
  arc A38 (27.9039, 33.0983) -> (27.8658, 33.0983) centre (27.8849, 33.0983) ccw
  arc A39 (27.8658, 32.8402) -> (27.9039, 32.8402) centre (27.8849, 32.8402) ccw
  line L20 (27.8849, 33.0983) -> (27.7558, 33.2274)
  arc A40 (27.7693, 33.2409) -> (27.7423, 33.2139) centre (27.7558, 33.2274) ccw
  arc A41 (27.8714, 33.0848) -> (27.8983, 33.1118) centre (27.8849, 33.0983) ccw
  line L21 (27.7558, 33.2274) -> (27.4977, 33.2274)
  arc A42 (27.4977, 33.2465) -> (27.4977, 33.2083) centre (27.4977, 33.2274) ccw
  arc A43 (27.7558, 33.2083) -> (27.7558, 33.2465) centre (27.7558, 33.2274) ccw
  line L22 (27.4977, 33.2274) -> (27.3686, 33.0983)
  arc A44 (27.3551, 33.1118) -> (27.3821, 33.0848) centre (27.3686, 33.0983) ccw
  arc A45 (27.5111, 33.2139) -> (27.4842, 33.2409) centre (27.4977, 33.2274) ccw
  line L23 (27.3686, 33.0983) -> (27.3686, 32.9692)
  arc A46 (27.3495, 32.9692) -> (27.3876, 32.9692) centre (27.3686, 32.9692) ccw
  arc A47 (27.3876, 33.0983) -> (27.3495, 33.0983) centre (27.3686, 33.0983) ccw
  line L24 (27.3686, 32.9692) -> (27.8849, 32.9692)
  arc A48 (27.8849, 32.9502) -> (27.8849, 32.9883) centre (27.8849, 32.9692) ccw
  arc A49 (27.3686, 32.9883) -> (27.3686, 32.9502) centre (27.3686, 32.9692) ccw
  line L25 (27.1022, 33.2274) -> (26.8441, 32.7111)
  arc A50 (26.827, 32.7196) -> (26.8611, 32.7026) centre (26.8441, 32.7111) ccw
  arc A51 (27.1193, 33.2189) -> (27.0852, 33.2359) centre (27.1022, 33.2274) ccw
  line L26 (26.8441, 32.7111) -> (26.5859, 33.2274)
  arc A52 (26.603, 33.2359) -> (26.5689, 33.2189) centre (26.5859, 33.2274) ccw
  arc A53 (26.827, 32.7026) -> (26.8611, 32.7196) centre (26.8441, 32.7111) ccw
  line L27 (26.3196, 32.7111) -> (26.3196, 32.8402)
  arc A54 (26.3386, 32.8402) -> (26.3005, 32.8402) centre (26.3196, 32.8402) ccw
  arc A55 (26.3005, 32.7111) -> (26.3386, 32.7111) centre (26.3196, 32.7111) ccw
  line L28 (26.3196, 32.8402) -> (26.1905, 32.8402)
  arc A56 (26.1905, 32.8592) -> (26.1905, 32.8211) centre (26.1905, 32.8402) ccw
  arc A57 (26.3196, 32.8211) -> (26.3196, 32.8592) centre (26.3196, 32.8402) ccw
  line L29 (26.1905, 32.8402) -> (26.1905, 32.7111)
  arc A58 (26.1714, 32.7111) -> (26.2095, 32.7111) centre (26.1905, 32.7111) ccw
  arc A59 (26.2095, 32.8402) -> (26.1714, 32.8402) centre (26.1905, 32.8402) ccw
  line L30 (26.1905, 32.7111) -> (26.3196, 32.7111)
  arc A60 (26.3196, 32.6921) -> (26.3196, 32.7302) centre (26.3196, 32.7111) ccw
  arc A61 (26.1905, 32.7302) -> (26.1905, 32.6921) centre (26.1905, 32.7111) ccw
  line L31 (25.1456, 33.2274) -> (24.8874, 33.4856)
  arc A62 (24.9009, 33.499) -> (24.8739, 33.4721) centre (24.8874, 33.4856) ccw
  arc A63 (25.1321, 33.2139) -> (25.159, 33.2409) centre (25.1456, 33.2274) ccw
  line L32 (24.8874, 33.4856) -> (24.8874, 32.7111)
  arc A64 (24.8684, 32.7111) -> (24.9065, 32.7111) centre (24.8874, 32.7111) ccw
  arc A65 (24.9065, 33.4856) -> (24.8684, 33.4856) centre (24.8874, 33.4856) ccw
  line L33 (25.1456, 32.7111) -> (24.6293, 32.7111)
  arc A66 (24.6293, 32.7302) -> (24.6293, 32.6921) centre (24.6293, 32.7111) ccw
  arc A67 (25.1456, 32.6921) -> (25.1456, 32.7302) centre (25.1456, 32.7111) ccw
  line L34 (24.3629, 32.8402) -> (24.2338, 32.7111)
  arc A68 (24.2203, 32.7246) -> (24.2473, 32.6976) centre (24.2338, 32.7111) ccw
  arc A69 (24.3764, 32.8267) -> (24.3494, 32.8537) centre (24.3629, 32.8402) ccw
  line L35 (24.2338, 32.7111) -> (23.9757, 32.7111)
  arc A70 (23.9757, 32.7302) -> (23.9757, 32.6921) centre (23.9757, 32.7111) ccw
  arc A71 (24.2338, 32.6921) -> (24.2338, 32.7302) centre (24.2338, 32.7111) ccw
  line L36 (23.9757, 32.7111) -> (23.8466, 32.8402)
  arc A72 (23.8601, 32.8537) -> (23.8331, 32.8267) centre (23.8466, 32.8402) ccw
  arc A73 (23.9622, 32.6976) -> (23.9891, 32.7246) centre (23.9757, 32.7111) ccw
  line L37 (23.8466, 32.8402) -> (23.8466, 33.3565)
  arc A74 (23.8656, 33.3565) -> (23.8275, 33.3565) centre (23.8466, 33.3565) ccw
  arc A75 (23.8275, 32.8402) -> (23.8656, 32.8402) centre (23.8466, 32.8402) ccw
  line L38 (23.8466, 33.3565) -> (23.9757, 33.4855)
  arc A76 (23.9891, 33.4721) -> (23.9622, 33.499) centre (23.9757, 33.4855) ccw
  arc A77 (23.8331, 33.37) -> (23.8601, 33.343) centre (23.8466, 33.3565) ccw
  line L39 (23.9757, 33.4855) -> (24.2338, 33.4855)
  arc A78 (24.2338, 33.4665) -> (24.2338, 33.5046) centre (24.2338, 33.4855) ccw
  arc A79 (23.9757, 33.5046) -> (23.9757, 33.4665) centre (23.9757, 33.4855) ccw
  line L40 (24.2338, 33.4855) -> (24.3629, 33.3565)
  arc A80 (24.3494, 33.343) -> (24.3764, 33.37) centre (24.3629, 33.3565) ccw
  arc A81 (24.2473, 33.499) -> (24.2203, 33.4721) centre (24.2338, 33.4855) ccw
  line L41 (24.3629, 33.3565) -> (24.3629, 33.2274)
  arc A82 (24.3438, 33.2274) -> (24.3819, 33.2274) centre (24.3629, 33.2274) ccw
  arc A83 (24.3819, 33.3565) -> (24.3438, 33.3565) centre (24.3629, 33.3565) ccw
  line L42 (24.3629, 33.2274) -> (24.2338, 33.0983)
  arc A84 (24.2203, 33.1118) -> (24.2473, 33.0848) centre (24.2338, 33.0983) ccw
  arc A85 (24.3764, 33.2139) -> (24.3494, 33.2409) centre (24.3629, 33.2274) ccw
  line L43 (24.2338, 33.0983) -> (23.8466, 33.0983)
  arc A86 (23.8466, 33.1174) -> (23.8466, 33.0793) centre (23.8466, 33.0983) ccw
  arc A87 (24.2338, 33.0793) -> (24.2338, 33.1174) centre (24.2338, 33.0983) ccw
  line L44 (31.5684, 35.1028) -> (31.5684, 36.2722)
  arc A88 (31.5938, 36.2722) -> (31.543, 36.2722) centre (31.5684, 36.2722) ccw
  arc A89 (31.543, 35.1028) -> (31.5938, 35.1028) centre (31.5684, 35.1028) ccw
  line L45 (31.9582, 36.2722) -> (31.1786, 36.2722)
  arc A90 (31.1786, 36.2976) -> (31.1786, 36.2468) centre (31.1786, 36.2722) ccw
  arc A91 (31.9582, 36.2468) -> (31.9582, 36.2976) centre (31.9582, 36.2722) ccw
  line L46 (30.7888, 36.2722) -> (30.7888, 35.2977)
  arc A92 (30.7634, 35.2977) -> (30.8142, 35.2977) centre (30.7888, 35.2977) ccw
  arc A93 (30.8142, 36.2722) -> (30.7634, 36.2722) centre (30.7888, 36.2722) ccw
  line L47 (30.7888, 35.2977) -> (30.5939, 35.1028)
  arc A94 (30.5759, 35.1208) -> (30.6119, 35.0848) centre (30.5939, 35.1028) ccw
  arc A95 (30.8068, 35.2797) -> (30.7708, 35.3157) centre (30.7888, 35.2977) ccw
  line L48 (30.5939, 35.1028) -> (30.2041, 35.1028)
  arc A96 (30.2041, 35.1282) -> (30.2041, 35.0774) centre (30.2041, 35.1028) ccw
  arc A97 (30.5939, 35.0774) -> (30.5939, 35.1282) centre (30.5939, 35.1028) ccw
  line L49 (30.2041, 35.1028) -> (30.0092, 35.2977)
  arc A98 (30.0272, 35.3157) -> (29.9913, 35.2797) centre (30.0092, 35.2977) ccw
  arc A99 (30.1861, 35.0848) -> (30.2221, 35.1208) centre (30.2041, 35.1028) ccw
  line L50 (30.0092, 35.2977) -> (30.0092, 36.2722)
  arc A100 (30.0346, 36.2722) -> (29.9838, 36.2722) centre (30.0092, 36.2722) ccw
  arc A101 (29.9838, 35.2977) -> (30.0346, 35.2977) centre (30.0092, 35.2977) ccw
  line L51 (29.6194, 35.1028) -> (29.6194, 36.2722)
  arc A102 (29.6448, 36.2722) -> (29.594, 36.2722) centre (29.6194, 36.2722) ccw
  arc A103 (29.594, 35.1028) -> (29.6448, 35.1028) centre (29.6194, 35.1028) ccw
  line L52 (29.6194, 36.2722) -> (29.0347, 36.2722)
  arc A104 (29.0347, 36.2976) -> (29.0347, 36.2468) centre (29.0347, 36.2722) ccw
  arc A105 (29.6194, 36.2468) -> (29.6194, 36.2976) centre (29.6194, 36.2722) ccw
  line L53 (29.0347, 36.2722) -> (28.8398, 36.0773)
  arc A106 (28.8218, 36.0953) -> (28.8578, 36.0593) centre (28.8398, 36.0773) ccw
  arc A107 (29.0527, 36.2542) -> (29.0168, 36.2901) centre (29.0347, 36.2722) ccw
  line L54 (28.8398, 36.0773) -> (28.8398, 35.6875)
  arc A108 (28.8144, 35.6875) -> (28.8652, 35.6875) centre (28.8398, 35.6875) ccw
  arc A109 (28.8652, 36.0773) -> (28.8144, 36.0773) centre (28.8398, 36.0773) ccw
  line L55 (28.8398, 35.6875) -> (29.0347, 35.4926)
  arc A110 (29.0168, 35.4746) -> (29.0527, 35.5105) centre (29.0347, 35.4926) ccw
  arc A111 (28.8578, 35.7055) -> (28.8218, 35.6695) centre (28.8398, 35.6875) ccw
  line L56 (29.0347, 35.4926) -> (29.6194, 35.4926)
  arc A112 (29.6194, 35.4672) -> (29.6194, 35.518) centre (29.6194, 35.4926) ccw
  arc A113 (29.0347, 35.518) -> (29.0347, 35.4672) centre (29.0347, 35.4926) ccw
  line L57 (29.2296, 35.4926) -> (28.8398, 35.1028)
  arc A114 (28.8218, 35.1208) -> (28.8578, 35.0848) centre (28.8398, 35.1028) ccw
  arc A115 (29.2476, 35.4746) -> (29.2117, 35.5105) centre (29.2296, 35.4926) ccw
  line L58 (24.9499, 33.9861) -> (24.4336, 34.5024)
  line L59 (29.9123, 34.7606) -> (30.4286, 34.7606)
  arc A116 (30.4286, 34.7415) -> (30.4286, 34.7796) centre (30.4286, 34.7606) ccw
  arc A117 (29.9123, 34.7796) -> (29.9123, 34.7415) centre (29.9123, 34.7606) ccw
  line L60 (30.4286, 34.7606) -> (30.4286, 34.3733)
  arc A118 (30.4095, 34.3733) -> (30.4476, 34.3733) centre (30.4286, 34.3733) ccw
  arc A119 (30.4476, 34.7606) -> (30.4095, 34.7606) centre (30.4286, 34.7606) ccw
  line L61 (30.4286, 34.3733) -> (30.1704, 34.5024)
  arc A120 (30.1789, 34.5194) -> (30.1619, 34.4854) centre (30.1704, 34.5024) ccw
  arc A121 (30.4201, 34.3563) -> (30.4371, 34.3904) centre (30.4286, 34.3733) ccw
  line L62 (30.1704, 34.5024) -> (30.0413, 34.5024)
  arc A122 (30.0413, 34.5214) -> (30.0413, 34.4833) centre (30.0413, 34.5024) ccw
  arc A123 (30.1704, 34.4833) -> (30.1704, 34.5214) centre (30.1704, 34.5024) ccw
  line L63 (30.0413, 34.5024) -> (29.9123, 34.3733)
  arc A124 (29.8988, 34.3868) -> (29.9257, 34.3599) centre (29.9123, 34.3733) ccw
  arc A125 (30.0548, 34.4889) -> (30.0279, 34.5159) centre (30.0414, 34.5024) ccw
  line L64 (29.9123, 34.3733) -> (29.9123, 34.1152)
  arc A126 (29.8932, 34.1152) -> (29.9313, 34.1152) centre (29.9123, 34.1152) ccw
  arc A127 (29.9313, 34.3733) -> (29.8932, 34.3733) centre (29.9123, 34.3733) ccw
  line L65 (29.9123, 34.1152) -> (30.0413, 33.9861)
  arc A128 (30.0279, 33.9726) -> (30.0548, 33.9996) centre (30.0414, 33.9861) ccw
  arc A129 (29.9257, 34.1286) -> (29.8988, 34.1017) centre (29.9123, 34.1152) ccw
  line L66 (30.0413, 33.9861) -> (30.2995, 33.9861)
  arc A130 (30.2995, 33.967) -> (30.2995, 34.0051) centre (30.2995, 33.9861) ccw
  arc A131 (30.0413, 34.0051) -> (30.0413, 33.967) centre (30.0413, 33.9861) ccw
  line L67 (30.2995, 33.9861) -> (30.4286, 34.1152)
  arc A132 (30.4421, 34.1017) -> (30.4151, 34.1286) centre (30.4286, 34.1152) ccw
  arc A133 (30.286, 33.9996) -> (30.313, 33.9726) centre (30.2995, 33.9861) ccw
  line L68 (28.8632, 34.1152) -> (28.7341, 33.9861)
  arc A134 (28.7207, 33.9996) -> (28.7476, 33.9726) centre (28.7341, 33.9861) ccw
  arc A135 (28.8767, 34.1017) -> (28.8498, 34.1286) centre (28.8632, 34.1152) ccw
  line L69 (28.7341, 33.9861) -> (28.6051, 33.9861)
  arc A136 (28.6051, 34.0052) -> (28.6051, 33.967) centre (28.6051, 33.9861) ccw
  arc A137 (28.7341, 33.967) -> (28.7341, 34.0052) centre (28.7341, 33.9861) ccw
  line L70 (28.6051, 33.9861) -> (28.476, 34.1152)
  arc A138 (28.4895, 34.1286) -> (28.4625, 34.1017) centre (28.476, 34.1152) ccw
  arc A139 (28.5916, 33.9726) -> (28.6186, 33.9996) centre (28.6051, 33.9861) ccw
  line L71 (28.476, 34.1152) -> (28.476, 34.7606)
  arc A140 (28.4951, 34.7606) -> (28.457, 34.7606) centre (28.476, 34.7606) ccw
  arc A141 (28.457, 34.1152) -> (28.4951, 34.1152) centre (28.476, 34.1152) ccw
  line L72 (28.6051, 34.7606) -> (28.3469, 34.7606)
  arc A142 (28.3469, 34.7796) -> (28.3469, 34.7415) centre (28.3469, 34.7606) ccw
  arc A143 (28.6051, 34.7415) -> (28.6051, 34.7796) centre (28.6051, 34.7606) ccw
  line L73 (28.0806, 34.5024) -> (28.0806, 34.1152)
  arc A144 (28.0615, 34.1152) -> (28.0996, 34.1152) centre (28.0806, 34.1152) ccw
  arc A145 (28.0996, 34.5024) -> (28.0615, 34.5024) centre (28.0806, 34.5024) ccw
  line L74 (28.0806, 34.1152) -> (27.9515, 33.9861)
  arc A146 (27.938, 33.9996) -> (27.965, 33.9726) centre (27.9515, 33.9861) ccw
  arc A147 (28.094, 34.1017) -> (28.0671, 34.1286) centre (28.0806, 34.1152) ccw
  line L75 (27.9515, 33.9861) -> (27.5643, 33.9861)
  arc A148 (27.5643, 34.0051) -> (27.5643, 33.967) centre (27.5643, 33.9861) ccw
  arc A149 (27.9515, 33.967) -> (27.9515, 34.0051) centre (27.9515, 33.9861) ccw
  line L76 (27.5643, 33.9861) -> (27.5643, 34.5024)
  arc A150 (27.5833, 34.5024) -> (27.5452, 34.5024) centre (27.5643, 34.5024) ccw
  arc A151 (27.5452, 33.9861) -> (27.5833, 33.9861) centre (27.5643, 33.9861) ccw
  line L77 (27.2979, 33.9861) -> (27.2979, 34.5024)
  arc A152 (27.317, 34.5024) -> (27.2789, 34.5024) centre (27.2979, 34.5024) ccw
  arc A153 (27.2789, 33.9861) -> (27.317, 33.9861) centre (27.2979, 33.9861) ccw
  line L78 (27.2979, 34.5024) -> (26.9107, 34.5024)
  arc A154 (26.9107, 34.5214) -> (26.9107, 34.4833) centre (26.9107, 34.5024) ccw
  arc A155 (27.2979, 34.4833) -> (27.2979, 34.5214) centre (27.2979, 34.5024) ccw
  line L79 (26.9107, 34.5024) -> (26.7816, 34.3733)
  arc A156 (26.7681, 34.3868) -> (26.7951, 34.3598) centre (26.7816, 34.3733) ccw
  arc A157 (26.9242, 34.4889) -> (26.8972, 34.5159) centre (26.9107, 34.5024) ccw
  line L80 (26.7816, 34.3733) -> (26.7816, 33.9861)
  arc A158 (26.7626, 33.9861) -> (26.8007, 33.9861) centre (26.7816, 33.9861) ccw
  arc A159 (26.8007, 34.3733) -> (26.7626, 34.3733) centre (26.7816, 34.3733) ccw
  line L81 (26.128, 33.9861) -> (26.3862, 33.9861)
  arc A160 (26.3862, 33.967) -> (26.3862, 34.0052) centre (26.3862, 33.9861) ccw
  arc A161 (26.128, 34.0051) -> (26.128, 33.967) centre (26.128, 33.9861) ccw
  line L82 (26.3862, 33.9861) -> (26.5152, 34.1152)
  arc A162 (26.5287, 34.1017) -> (26.5018, 34.1286) centre (26.5152, 34.1152) ccw
  arc A163 (26.3727, 33.9996) -> (26.3996, 33.9726) centre (26.3862, 33.9861) ccw
  line L83 (26.5152, 34.1152) -> (26.5152, 34.3733)
  arc A164 (26.5343, 34.3733) -> (26.4962, 34.3733) centre (26.5152, 34.3733) ccw
  arc A165 (26.4962, 34.1152) -> (26.5343, 34.1152) centre (26.5152, 34.1152) ccw
  line L84 (26.5152, 34.3733) -> (26.3861, 34.5024)
  arc A166 (26.3996, 34.5159) -> (26.3727, 34.4889) centre (26.3862, 34.5024) ccw
  arc A167 (26.5018, 34.3598) -> (26.5287, 34.3868) centre (26.5152, 34.3733) ccw
  line L85 (26.3861, 34.5024) -> (26.128, 34.5024)
  arc A168 (26.128, 34.5214) -> (26.128, 34.4833) centre (26.128, 34.5024) ccw
  arc A169 (26.3861, 34.4833) -> (26.3861, 34.5214) centre (26.3861, 34.5024) ccw
  line L86 (26.128, 34.5024) -> (25.9989, 34.3733)
  arc A170 (25.9855, 34.3868) -> (26.0124, 34.3598) centre (25.9989, 34.3733) ccw
  arc A171 (20.6794, 36.2722) -> (20.6286, 36.2722) centre (20.654, 36.2722) ccw
  arc A172 (20.6286, 35.1028) -> (20.6794, 35.1028) centre (20.654, 35.1028) ccw
  line L87 (20.654, 36.2722) -> (20.654, 35.1028)
  arc A173 (21.4336, 35.6621) -> (21.4336, 35.7129) centre (21.4336, 35.6875) ccw
  arc A174 (20.654, 35.7129) -> (20.654, 35.6621) centre (20.654, 35.6875) ccw
  line L88 (21.4336, 35.6875) -> (20.654, 35.6875)
  arc A175 (21.4082, 35.1028) -> (21.459, 35.1028) centre (21.4336, 35.1028) ccw
  arc A176 (21.459, 36.2722) -> (21.4082, 36.2722) centre (21.4336, 36.2722) ccw
  line L89 (21.4336, 35.1028) -> (21.4336, 36.2722)
  arc A177 (22.0004, 35.0848) -> (22.0363, 35.1208) centre (22.0183, 35.1028) ccw
  arc A178 (21.8414, 35.3157) -> (21.8055, 35.2797) centre (21.8234, 35.2977) ccw